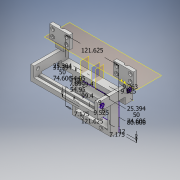
# Autodesk Inventor part: rearChassis_final
Saved by Autodesk Inventor 2018 (Build 220112000, 112)
## iProperties
Created: 2017-10-21
Part Number: rearChassis_final
Material: Generic
Document SubType Name: Modeling
Designer: Prakash
Density: 1 g/cm^3
Appearance: Default
d0: 1.500 mm
d1: 10.000 mm
d2: 18.000 mm
d3: 18.000 mm
d4: 30.000 mm
d5: 0.00 deg
d8: 10.000 mm
d9: 0.00 deg
d10: 3.588 mm
d11: 3.588 mm
d12: 34.763 mm
d13: 0.00 deg
d15: 9.763 mm
d16: 9.525 mm
d17: 8.000 mm
d22: 10.000 mm
d25: 10.000 mm
d26: 5.000 mm
d27: 70.000 mm
d28: 0.00 deg
d74: 7.000 mm
d75: 7.000 mm
d76: 7.500 mm
d77: 7.500 mm
d79: 7.500 mm
d80: 7.500 mm
d81: 3.000 mm
d89: 8.000 mm
d90: 3.175 mm
d91: 0.00 deg
d104: -68.000 mm
d117: 45.250 mm
Author: Prakash
Autodesk Inventor part; units mm, degrees
ref_plane "YZ Plane" through (0, 0, 0) normal (1, 0, 0) x (0, 1, 0)
ref_plane "XZ Plane" through (0, 0, 0) normal (0, 1, 0) x (-1, 0, 0)
ref_plane "XY Plane" through (0, 0, 0) normal (0, 0, 1) x (1, 0, 0)
sketch "Sketch1" plane through (0, 0, 0) normal (0, 0, 1) x (1, 0, 0)
  line L0 (0, 0) -> (45.5394, 0)
  line L1 (45.5394, 0) -> (45.5394, 7.5)
  line L2 (45.5394, 7.5) -> (27.5394, 7.5)
  line L3 (0, 7.5) -> (0, 0)
  line L4 (22.7697, 7.5) -> (22.7697, 9) construction
  arc A0 (18, 7.5) -> (27.5394, 7.5) centre (22.7697, 9) ccw
  circle A1 centre (22.7697, 9) radius 9 construction
  line L5 (18, 7.5) -> (0, 7.5)
  line L6 (27.5394, 7.5) -> (22.7697, 7.5) construction
  line L7 (22.7697, 7.5) -> (18, 7.5) construction
  dimension "d0" = 1.5
  dimension "d1" = 10
  dimension "d2" = 18
  dimension "d3" = 18
  constraints: 16 end point, 5 parallel, 2 centre point, 2 coincident, 2 point on circle, 1 collinear, 1 horizontal, 1 perpendicular, 1 tangent, 1 vertical
  measures "d0" distance of L4.start L4.end
  measures "d1" diameter of A0
  measures "d2" distance of L1.end L2.end
  measures "d3" diameter of A1
extrude "Extrusion1" add sketch "Sketch1" along normal blind 30
sketch "Sketch3" plane through (0, 0, 0) normal (0, 0, -1) x (-1, 0, 0)
  circle A0 centre (-22.7697, 9) radius 9 construction
  arc A1 (-27.5394, 7.5) -> (-18, 7.5) centre (-22.7697, 9) ccw projected
  arc A2 (-27.5394, 7.5) -> (-18, 7.5) centre (-22.7697, 9) ccw projected
  arc A3 (-27.5394, 7.5) -> (-18, 7.5) centre (-22.7697, 9) ccw projected
  circle A4 centre (-22.7697, 9) radius 5
  line L0 (-31.7697, 9) -> (-31.7697, 0)
  line L1 (-13.7697, 9) -> (-13.7697, 0)
  arc A5 (-22.7697, 0) -> (-13.7697, 9) centre (-22.7697, 9) ccw
  line L2 (0, 0) -> (-45.5394, 0) projected
  line L3 (-31.7697, 0) -> (-22.7697, 0)
  line L4 (-22.7697, 0) -> (-13.7697, 0)
  arc A6 (-31.7697, 9) -> (-22.7697, 0) centre (-22.7697, 9) ccw
  arc A7 (-13.7697, 9) -> (-31.7697, 9) centre (-22.7697, 9) ccw
  constraints: 8 end point, 8 point on circle, 3 centre point, 2 coincident, 2 collinear, 2 point on line, 2 tangent, 2 vertical, 1 concentric, 3 other
extrude "Extrusion2" add sketch "Sketch3" along normal blind 10
sketch "Sketch5" plane through (0, 0, -10) normal (0, 0, -1) x (-1, 0, 0)
  line L0 (-31.7697, 0) -> (-13.7697, 0) projected
  line L1 (-22.7697, 0) -> (-19.1822, 0)
  line L2 (-22.7697, 0) -> (-26.3572, 0)
  line L3 (-26.3572, 0) -> (-19.1822, 0)
  line L4 (-19.1822, 0) -> (-19.1822, 18)
  line L5 (-19.1822, 18) -> (-26.3572, 18)
  line L6 (-26.3572, 18) -> (-26.3572, 0)
  arc A0 (-13.7697, 9) -> (-31.7697, 9) centre (-22.7697, 9) ccw projected
  point P0 (0, 0)
  dimension "d10" = 3.5875
  dimension "d11" = 3.5875
  constraints: 12 end point, 2 parallel, 2 point on line, 1 horizontal, 1 midpoint, 1 perpendicular, 1 tangent
  measures "d10" distance of L1.start L1.end
  measures "d11" distance of L1.start L2.end
extrude "Extrusion3" add sketch "Sketch5" along normal blind 34.763
sketch "Sketch6" plane through (26.3572, 5.5172, -10) normal (1, 0, 0) x (0, 0, -1)
  line L0 (-10, 3.4828) -> (0, 3.4828) projected
  line L1 (0, 3.4828) -> (9.763, 3.4828) construction
  circle A0 centre (9.763, 3.4828) radius 4.7625
  circle A1 centre (9.763, 3.4828) radius 4
  point P0 (-10, -5.5172)
  dimension "d15" = 9.763
  dimension "d16" = 9.525
  dimension "d17" = 8
  constraints: 2 centre point, 2 coincident, 2 end point, 1 horizontal
  measures "d15" distance of L0.end L1.end
  measures "d16" diameter of A0
  measures "d17" diameter of A1
sketch "Sketch7" plane through (19.1822, 5.5172, -10) normal (-1, 0, 0) x (0, 0, 1)
  circle A0 centre (-9.763, 3.4828) radius 4 projected
  circle A1 centre (-9.763, 3.4828) radius 4.7625 projected
  point P0 (10, -5.5172)
sketch "Sketch8" plane through (19.1822, 5.5172, -10) normal (-1, 0, 0) x (0, 0, 1)
  line L0 (-34.763, -5.5172) -> (-34.763, 12.4828) projected
  line L1 (-34.763, 12.4828) -> (-24.763, 12.4828)
  line L2 (-24.763, 12.4828) -> (-24.763, 5.9828)
  line L3 (-24.763, 5.9828) -> (-34.763, 5.9828)
  line L4 (-34.763, 5.9828) -> (-34.763, 12.4828)
  line L5 (-34.763, -5.5172) -> (-24.763, -5.5172)
  line L6 (-24.763, -5.5172) -> (-24.763, 0.9828)
  line L7 (-24.763, 0.9828) -> (-34.763, 0.9828)
  line L8 (-34.763, 0.9828) -> (-34.763, -5.5172)
  point P0 (10, -5.5172)
  dimension "d22" = 10
  dimension "d25" = 10
  dimension "d26" = 5
  constraints: 16 end point, 4 parallel, 2 horizontal, 2 perpendicular, 1 collinear
  measures "d22" distance of L2.end L3.end
  measures "d25" distance of L6.end L7.end
  measures "d26" distance between parallel lines of L7 L3
extrude "Extrusion6" add sketch "Sketch8" along normal blind 70
sketch "Sketch11" plane through (0, 7.5, 30) normal (0, 1, 0) x (1, 0, 0)
  line L0 (13.7697, 30) -> (0, 30) projected
  line L1 (7, 30) -> (7, 0)
  line L2 (18, 0) -> (0, 0) projected
  line L3 (38.5394, 30) -> (38.5394, 0)
  line L4 (0, 30) -> (0, 0) projected
  line L5 (45.5394, 30) -> (45.5394, 0) projected
  line L6 (45.5394, 30) -> (31.7697, 30) projected
  line L7 (45.5394, 0) -> (27.5394, 0) projected
  point P0 (7, 22.5)
  point P1 (7, 7.5)
  point P2 (38.5394, 22.5)
  point P3 (38.5394, 7.5)
  dimension "d74" = 7
  dimension "d75" = 7
  dimension "d76" = 7.5
  dimension "d77" = 7.5
  dimension "d79" = 7.5
  dimension "d80" = 7.5
  constraints: 8 point on line, 4 end point, 2 vertical
  measures "d74" distance between parallel lines of L4 L1
  measures "d75" distance between parallel lines of L5 L3
  measures "d76" distance of L1.start point (7, 22.5)
  measures "d77" distance of L1.end point (7, 7.5)
  measures "d79" distance of L3.start point (38.539, 22.5)
  measures "d80" distance of L3.end point (38.539, 7.5)
hole "Hole3" at (7, 7.5, 7.5) at (7, 7.5, 22.5) at (38.5394, 7.5, 7.5) at (38.5394, 7.5, 22.5) direction (0, -1, 0) diameter 3 end up to face face through (19.7697, 0, 20) facing (0, -1, 0)
sketch "Sketch13" plane through (0, 0, 30) normal (0, -1, 0) x (1, 0, 0)
  circle A0 centre (7, -7.5) radius 1.5 projected
  circle A1 centre (38.5394, -7.5) radius 1.5 projected
  circle A2 centre (38.5394, -22.5) radius 1.5 projected
  circle A3 centre (7, -22.5) radius 1.5 projected
  line L0 (11, -9.8094) -> (7, -12.1188)
  line L1 (7, -12.1188) -> (3, -9.8094)
  line L2 (3, -9.8094) -> (3, -5.1906)
  line L3 (3, -5.1906) -> (7, -2.8812)
  line L4 (7, -2.8812) -> (11, -5.1906)
  line L5 (11, -5.1906) -> (11, -9.8094)
  line L6 (11, -20.1906) -> (11, -24.8094)
  line L7 (11, -24.8094) -> (7, -27.1188)
  line L8 (7, -27.1188) -> (3, -24.8094)
  line L9 (3, -24.8094) -> (3, -20.1906)
  line L10 (3, -20.1906) -> (7, -17.8812)
  line L11 (7, -17.8812) -> (11, -20.1906)
  line L12 (42.5394, -20.1906) -> (42.5394, -24.8094)
  line L13 (42.5394, -24.8094) -> (38.5394, -27.1188)
  line L14 (38.5394, -27.1188) -> (34.5394, -24.8094)
  line L15 (34.5394, -24.8094) -> (34.5394, -20.1906)
  line L16 (34.5394, -20.1906) -> (38.5394, -17.8812)
  line L17 (38.5394, -17.8812) -> (42.5394, -20.1906)
  line L18 (38.5394, -2.8812) -> (42.5394, -5.1906)
  line L19 (42.5394, -5.1906) -> (42.5394, -9.8094)
  line L20 (42.5394, -9.8094) -> (38.5394, -12.1188)
  line L21 (38.5394, -12.1188) -> (34.5394, -9.8094)
  line L22 (34.5394, -9.8094) -> (34.5394, -5.1906)
  line L23 (34.5394, -5.1906) -> (38.5394, -2.8812)
  line L24 (0, -30) -> (0, 0) projected
  line L25 (45.5394, -30) -> (45.5394, 0) projected
  point P0 (38.5394, -22.5)
  point P1 (38.5394, -7.5)
  dimension "d89" = 8
  constraints: 48 end point, 4 coincident, 4 parallel, 3 equal length, 52 other
  measures "d89" distance between parallel lines of L0 L3
extrude "Extrusion7" cut sketch "Sketch13" against normal blind 3.175
mirror "Mirror1" about plane through (-50.8178, 14.75, -39.763) normal (-1, 0, 0) of "Extrusion6", "Extrusion3", "Extrusion2", "Extrusion1", "Hole3", "Extrusion7"
ref_plane "Work Plane1" through (-41.6428, 5.5172, -10) normal (1, 0, 0) x (0, 0, -1)
ref_plane "Work Plane2" through (-75.5678, 5.5172, -10) normal (1, 0, 0) x (0, 0, -1)
ref_plane "Work Plane4" through (-133.4053, 9, 0) normal (0, 0, 1) x (1, 0, 0)
split body "Split1" result two bodies by plane through (-133.4053, 9, 0) normal (0, 0, 1) first body at (-120.4821, 0.5, 13.2698) (18.8465, 0.5, 16.7302)
ref_plane "Halfway plane" through (-50.8178, 5.5172, -10) normal (-1, 0, 0) x (0, 0, 1)
sketch "Sketch26" plane through (26.3572, 18, -10) normal (0, 1, 0) x (1, 0, 0)
  line L0 (0, 34.763) -> (-154.35, 34.763) projected
  line L1 (-154.35, 0) -> (-154.35, 34.763) projected
  line L2 (-121.625, 84.763) -> (-121.625, 34.763)
  line L3 (-7.175, 34.763) -> (-147.175, 34.763) projected
  line L4 (-32.725, 84.763) -> (-32.725, 34.763)
  line L5 (-32.725, 54.157) -> (-121.625, 54.157)
  line L6 (-121.625, 54.157) -> (-121.625, 66.157)
  line L7 (-121.625, 66.157) -> (-32.725, 66.157)
  line L8 (-32.725, 66.157) -> (-32.725, 54.157)
  line L9 (-32.725, 54.157) -> (-121.625, 66.157) construction
  line L10 (-121.625, 54.157) -> (-32.725, 66.157) construction
  line L11 (-121.625, 103.369) -> (-32.725, 103.369)
  line L12 (-32.725, 103.369) -> (-32.725, 115.369)
  line L13 (-32.725, 115.369) -> (-121.625, 115.369)
  line L14 (-121.625, 115.369) -> (-121.625, 103.369)
  line L15 (-121.625, 103.369) -> (-32.725, 115.369) construction
  line L16 (-32.725, 103.369) -> (-121.625, 115.369) construction
  line L17 (-121.625, 84.763) -> (-121.625, 103.369)
  line L18 (-32.725, 84.763) -> (-32.725, 103.369)
  line L19 (-121.625, 34.763) -> (-114.45, 34.763)
  line L20 (-114.45, 34.763) -> (-114.45, 115.369)
  line L21 (-114.45, 115.369) -> (-121.625, 115.369)
  line L22 (-121.625, 115.369) -> (-121.625, 34.763)
  line L23 (-32.725, 34.763) -> (-39.9, 34.763)
  line L24 (-39.9, 34.763) -> (-39.9, 115.369)
  line L25 (-39.9, 115.369) -> (-32.725, 115.369)
  line L26 (-32.725, 115.369) -> (-32.725, 34.763)
  line L27 (-121.625, 103.369) -> (-32.725, 103.369)
  line L28 (-32.725, 103.369) -> (-32.725, 115.369)
  line L29 (-32.725, 115.369) -> (-121.625, 115.369)
  line L30 (-121.625, 115.369) -> (-121.625, 103.369)
  point P0 (-26.3572, -10)
  point P1 (-77.175, 60.157)
  point P2 (-77.175, 109.369)
  point P3 (-99.4, 60.157)
  point P4 (-54.95, 60.157)
  point P5 (-54.95, 109.369)
  point P6 (-99.4, 109.369)
  dimension "d149" = 12
  dimension "d150" = 12
  dimension "d153" = 121.625
  dimension "d154" = 7.175
  dimension "d155" = 7.175
  dimension "d156" = 7.688
  dimension "d157" = 80.606
  dimension "d158" = 31.394
  dimension "d159" = 121.625
  dimension "d160" = 50
  dimension "d161" = 74.606
  dimension "d162" = 99.4
  dimension "d163" = 25.394
  dimension "d164" = 99.4
  dimension "d165" = 74.606
  dimension "d166" = 54.95
  dimension "d167" = 25.394
  dimension "d168" = 54.95
  dimension "d169" = 50
  constraints: 56 end point, 15 parallel, 5 perpendicular, 4 midpoint, 4 point on line, 3 horizontal, 1 collinear, 1 vertical
  measures "d149" distance of L5.end L6.end
  measures "d150" distance of L12.end L11.end
  measures "d153" distance between parallel lines of L18 L1
  measures "d154" distance of L21.end L20.end
  measures "d155" distance of L24.end L25.end
  measures "d156" angle of L3 L15
  measures "d157" distance between parallel lines of L3 L13
  measures "d158" distance between parallel lines of L3 L7
  measures "d159" distance between parallel lines of L8 L1
  measures "d160" distance from line of L4.start L3
  measures "d161" distance from line of point (-54.95, 109.369) L3
  measures "d162" distance from line of point (-54.95, 109.369) L1
  measures "d163" distance from line of point (-54.95, 60.157) L3
  measures "d164" distance from line of point (-54.95, 60.157) L1
  measures "d165" distance from line of point (-99.4, 109.369) L3
  measures "d166" distance from line of point (-99.4, 109.369) L1
  measures "d167" distance from line of point (-99.4, 60.157) L3
  measures "d168" distance from line of point (-99.4, 60.157) L1
  measures "d169" distance from line of L2.start L3
extrude "Extrusion14" add sketch "Sketch26" against normal up to surface (18 mm away) contours L0 L24 L5 L4 | L5 L24 L7 L4 | L0 L2 L5 L20 | L5 L20 L7 L24 | L7 L24 L11 L18 L4 | L5 L2 L7 L20 | L7 L2 L17 L11 L20 | L24 L13 L12 L11 | L11 L20 L13 L24 | L11 L14 L13 L20 bodies 3
hole "Hole5" at (-28.5928, 18, -70.157) at (-28.5928, 18, -119.369) at (-73.0428, 18, -70.157) at (-73.0428, 18, -119.369) direction (0, -1, 0) diameter 3 end up to face face through (-65.6345, 0, -38.0963) facing (0, -1, 0) bodies 3
sketch "Sketch27" plane through (13.7697, 0, 0) normal (0, -1, 0) x (1, 0, 0)
  line L0 (-2.7697, 9.8094) -> (-2.7697, 5.1906) projected
  line L1 (-6.7697, 12.1188) -> (-2.7697, 9.8094) projected
  line L2 (-13.7697, 0) -> (31.7697, 0) projected
  line L3 (31.7697, 0) -> (31.7697, 30) projected
  line L4 (-13.7697, 30) -> (31.7697, 30) projected
  line L5 (-13.7697, 0) -> (-13.7697, 30) projected
  line L6 (20.7697, 24.8094) -> (24.7697, 27.1188) projected
  line L7 (24.7697, 27.1188) -> (28.7697, 24.8094) projected
  line L8 (28.7697, 24.8094) -> (28.7697, 20.1906) projected
  line L9 (28.7697, 20.1906) -> (24.7697, 17.8812) projected
  line L10 (24.7697, 17.8812) -> (20.7697, 20.1906) projected
  line L11 (20.7697, 20.1906) -> (20.7697, 24.8094) projected
  line L12 (-6.7697, 12.1188) -> (-2.7697, 9.8094) projected
  line L13 (-2.7697, 9.8094) -> (-2.7697, 5.1906) projected
  line L14 (-2.7697, 5.1906) -> (-6.7697, 2.8812) projected
  line L15 (-6.7697, 2.8812) -> (-10.7697, 5.1906) projected
  line L16 (-10.7697, 5.1906) -> (-10.7697, 9.8094) projected
  line L17 (-10.7697, 9.8094) -> (-6.7697, 12.1188) projected
  line L18 (-2.7697, 24.8094) -> (-2.7697, 20.1906) projected
  line L19 (-2.7697, 20.1906) -> (-6.7697, 17.8812) projected
  line L20 (-6.7697, 17.8812) -> (-10.7697, 20.1906) projected
  line L21 (-10.7697, 20.1906) -> (-10.7697, 24.8094) projected
  line L22 (-10.7697, 24.8094) -> (-6.7697, 27.1188) projected
  line L23 (-6.7697, 27.1188) -> (-2.7697, 24.8094) projected
  line L24 (24.7697, 12.1188) -> (28.7697, 9.8094) projected
  line L25 (28.7697, 9.8094) -> (28.7697, 5.1906) projected
  line L26 (28.7697, 5.1906) -> (24.7697, 2.8812) projected
  line L27 (24.7697, 2.8812) -> (20.7697, 5.1906) projected
  line L28 (20.7697, 5.1906) -> (20.7697, 9.8094) projected
  line L29 (20.7697, 9.8094) -> (24.7697, 12.1188) projected
  circle A0 centre (-42.3625, -70.157) radius 1.5 projected
  line L30 (-44.6719, -74.157) -> (-46.9813, -70.157)
  line L31 (-46.9813, -70.157) -> (-44.6719, -66.157)
  line L32 (-44.6719, -66.157) -> (-40.0531, -66.157)
  line L33 (-40.0531, -66.157) -> (-37.7437, -70.157)
  line L34 (-37.7437, -70.157) -> (-40.0531, -74.157)
  line L35 (-40.0531, -74.157) -> (-44.6719, -74.157)
  circle A1 centre (-86.8125, -70.157) radius 1.5 projected
  line L36 (-91.4313, -70.157) -> (-89.1219, -66.157)
  line L37 (-89.1219, -66.157) -> (-84.5031, -66.157)
  line L38 (-84.5031, -66.157) -> (-82.1937, -70.157)
  line L39 (-82.1937, -70.157) -> (-84.5031, -74.157)
  line L40 (-84.5031, -74.157) -> (-89.1219, -74.157)
  line L41 (-89.1219, -74.157) -> (-91.4313, -70.157)
  circle A2 centre (-86.8125, -119.369) radius 1.5 projected
  line L42 (-91.4313, -119.369) -> (-89.1219, -115.369)
  line L43 (-89.1219, -115.369) -> (-84.5031, -115.369)
  line L44 (-84.5031, -115.369) -> (-82.1937, -119.369)
  line L45 (-82.1937, -119.369) -> (-84.5031, -123.369)
  line L46 (-84.5031, -123.369) -> (-89.1219, -123.369)
  line L47 (-89.1219, -123.369) -> (-91.4313, -119.369)
  circle A3 centre (-42.3625, -119.369) radius 1.5 projected
  line L48 (-46.9813, -119.369) -> (-44.6719, -115.369)
  line L49 (-44.6719, -115.369) -> (-40.0531, -115.369)
  line L50 (-40.0531, -115.369) -> (-37.7437, -119.369)
  line L51 (-37.7437, -119.369) -> (-40.0531, -123.369)
  line L52 (-40.0531, -123.369) -> (-44.6719, -123.369)
  line L53 (-44.6719, -123.369) -> (-46.9813, -119.369)
  point P0 (-42.3625, -70.157)
  point P1 (-86.8125, -70.157)
  point P2 (-86.8125, -119.369)
  point P3 (-42.3625, -119.369)
  constraints: 48 end point, 4 coincident, 4 equal length, 4 horizontal, 52 other
extrude "Extrusion15" cut sketch "Sketch27" against normal blind 3.175 contours L30 L31 L32 L33 L34 L35 | L36 L37 L38 L39 L40 L41 | L42 L43 L44 L45 L46 L47 | L48 L49 L50 L51 L52 L53 bodies 3
sketch "Sketch30" plane through (13.7697, 0, 0) normal (0, -1, 0) x (1, 0, 0)
  line L0 (12.5875, -10) -> (12.5875, -44.763) projected
  line L1 (5.4125, -10) -> (12.5875, -10)
  line L2 (12.5875, -10) -> (12.5875, -29.526)
  line L3 (12.5875, -29.526) -> (5.4125, -29.526)
  line L4 (5.4125, -29.526) -> (5.4125, -10)
  line L5 (-141.7625, -10) -> (-134.5875, -10) projected
  line L6 (-141.7625, -10) -> (-134.5875, -10)
  line L7 (-134.5875, -10) -> (-134.5875, -29.526)
  line L8 (-134.5875, -29.526) -> (-141.7625, -29.526)
  line L9 (-141.7625, -29.526) -> (-141.7625, -10)
  point P0 (-13.7697, 0)
  dimension "d181" = 19.526
  dimension "d182" = 19.526
  constraints: 16 end point, 5 equal length, 2 perpendicular, 1 horizontal
  measures "d181" distance of L0.start L2.end
  measures "d182" distance of L5.end L7.end
extrude "Extrusion16" add sketch "Sketch30" along normal blind 62.5 bodies 3
sketch "Sketch31" plane through (26.3572, 5.5172, -10) normal (1, 0, 0) x (0, 0, -1)
  line L0 (19.526, -68.0172) -> (0, -68.0172) construction
  line L1 (9.763, -68.0172) -> (9.763, -59.0172) construction
  circle A0 centre (9.763, -59.0172) radius 4.7625
  circle A1 centre (9.763, -59.0172) radius 4
  point P0 (-10, -5.5172)
  dimension "d185" = 9
  dimension "d186" = 9.525
  dimension "d187" = 8
  constraints: 2 centre point, 2 coincident, 2 end point, 1 midpoint, 1 vertical
  measures "d185" distance of L1.start L1.end
  measures "d186" diameter of A0
  measures "d187" diameter of A1
extrude "Extrusion17" cut sketch "Sketch31" against normal up to surface (7.175 mm away) contours A1 bodies 3
extrude "Extrusion18" cut sketch "Sketch31" against normal blind 3.175 bodies 3
mirror "Mirror4" about plane through (-50.8178, 5.5172, -10) normal (-1, 0, 0) of "Extrusion18", "Extrusion17" bodies 3
sketch "Sketch35" plane through (19.1822, 6.5, -34.763) normal (0, 1, 0) x (1, 0, 0)
  line L0 (-94.5344, 88.606) -> (-96.8438, 84.606) projected
  line L1 (-96.8438, 84.606) -> (-94.5344, 80.606) projected
  line L2 (-94.5344, 80.606) -> (-89.9156, 80.606) projected
  line L3 (-89.9156, 80.606) -> (-87.6062, 84.606) projected
  line L4 (-87.6062, 84.606) -> (-89.9156, 88.606) projected
  line L5 (-89.9156, 88.606) -> (-94.5344, 88.606) projected
  line L6 (-45.4656, 39.394) -> (-50.0844, 39.394) projected
  line L7 (-50.0844, 39.394) -> (-52.3938, 35.394) projected
  line L8 (-52.3938, 35.394) -> (-50.0844, 31.394) projected
  line L9 (-50.0844, 31.394) -> (-45.4656, 31.394) projected
  line L10 (-45.4656, 31.394) -> (-43.1562, 35.394) projected
  line L11 (-43.1562, 35.394) -> (-45.4656, 39.394) projected
  line L12 (-94.5344, 39.394) -> (-96.8438, 35.394) projected
  line L13 (-96.8438, 35.394) -> (-94.5344, 31.394) projected
  line L14 (-94.5344, 31.394) -> (-89.9156, 31.394) projected
  line L15 (-89.9156, 31.394) -> (-87.6062, 35.394) projected
  line L16 (-87.6062, 35.394) -> (-89.9156, 39.394) projected
  line L17 (-89.9156, 39.394) -> (-94.5344, 39.394) projected
  line L18 (-50.0844, 88.606) -> (-52.3938, 84.606) projected
  line L19 (-52.3938, 84.606) -> (-50.0844, 80.606) projected
  line L20 (-50.0844, 80.606) -> (-45.4656, 80.606) projected
  line L21 (-45.4656, 80.606) -> (-43.1562, 84.606) projected
  line L22 (-43.1562, 84.606) -> (-45.4656, 88.606) projected
  line L23 (-45.4656, 88.606) -> (-50.0844, 88.606) projected
  line L24 (7.175, -5.237) -> (0, -5.237) projected
  line L25 (0, -5.237) -> (0, 0) projected
  line L26 (0, 0) -> (-140, 0) projected
  line L27 (-140, -5.237) -> (-140, 0) projected
  line L28 (-140, -5.237) -> (-147.175, -5.237) projected
  line L29 (-147.175, -5.237) -> (-147.175, 10) projected
  line L30 (-114.45, 10) -> (-147.175, 10) projected
  line L31 (-114.45, 90.606) -> (-114.45, 10) projected
  line L32 (-25.55, 90.606) -> (-114.45, 90.606) projected
  line L33 (-25.55, 10) -> (-25.55, 90.606) projected
  line L34 (7.175, 10) -> (-25.55, 10) projected
  line L35 (7.175, -5.237) -> (7.175, 10) projected
  line L36 (-32.725, 41.394) -> (-107.275, 41.394) projected
  line L37 (-32.725, 78.606) -> (-32.725, 41.394) projected
  line L38 (-107.275, 78.606) -> (-32.725, 78.606) projected
  line L39 (-107.275, 41.394) -> (-107.275, 78.606) projected
  line L40 (-32.725, 29.394) -> (-32.725, 10) projected
  line L41 (-107.275, 29.394) -> (-32.725, 29.394) projected
  line L42 (-107.275, 10) -> (-107.275, 29.394) projected
  line L43 (-32.725, 10) -> (-107.275, 10) projected
  line L44 (0, 0) -> (0, 10)
  line L45 (0, 10) -> (-140, 10)
  line L46 (-140, 10) -> (-140, 0)
  line L47 (-140, 0) -> (0, 0)
  point P0 (-19.1822, -34.763)
  dimension "d192" = 140
  constraints: 8 end point, 2 parallel, 2 perpendicular, 1 point on line
  measures "d192" distance between parallel lines of L44 L46
extrude "Extrusion19" add sketch "Sketch35" along normal up to next contours L26 L46 L30 L45 L43 L34 L44 bodies 3
sketch "Sketch36" plane through (26.3572, 0, -29.526) normal (0, 0, -1) x (-1, 0, 0)
  line L0 (0, 0) -> (7.175, 0) projected
  line L1 (0, 0) -> (0, -62.5) projected
  line L2 (7.175, -62.5) -> (0, -62.5) projected
  line L3 (7.175, 0) -> (7.175, -62.5) projected
  line L4 (147.175, 0) -> (154.35, 0) projected
  line L5 (147.175, 0) -> (147.175, -62.5) projected
  line L6 (154.35, -62.5) -> (147.175, -62.5) projected
  line L7 (154.35, 0) -> (154.35, -62.5) projected
  line L8 (7.175, -62.5) -> (0, -62.5)
  line L9 (0, -62.5) -> (0, -44.5)
  line L10 (0, -44.5) -> (7.175, -44.5)
  line L11 (7.175, -44.5) -> (7.175, -62.5)
  point P0 (26.3572, 0)
  dimension "d195" = 18
  constraints: 8 end point, 2 parallel, 1 horizontal, 1 perpendicular
  measures "d195" distance of L1.end L9.end
extrude "Extrusion20" add sketch "Sketch36" along normal blind 14 contours L10 L3 L2 L1 bodies 3
sketch "Sketch37" plane through (19.1822, 5.5172, -10) normal (-1, 0, 0) x (0, 0, 1)
  line L0 (-24.763, 12.4828) -> (-24.763, -5.5172) projected
  line L1 (-19.526, -5.5172) -> (-24.763, -5.5172) projected
  line L2 (-19.526, -5.5172) -> (-19.526, -50.0172) projected
  line L3 (-19.526, -50.0172) -> (-33.526, -50.0172) projected
  line L4 (-33.526, -68.0172) -> (-33.526, -50.0172) projected
  line L5 (0, -68.0172) -> (-33.526, -68.0172) projected
  line L6 (0, -5.5172) -> (0, -68.0172) projected
  line L7 (0, 0) -> (0, -5.5172) projected
  line L8 (0, 0) -> (0, 6.9656) projected
  line L9 (0, 11.7369) -> (0, 6.9656) projected
  line L10 (0, 11.7369) -> (0, 12.4828) projected
  line L11 (0, 12.4828) -> (-24.763, 12.4828) projected
  circle A0 centre (-9.763, -59.0172) radius 4 projected
  line L12 (-33.526, -50.0172) -> (-23.526, -50.0172)
  line L13 (-23.526, -50.0172) -> (-23.526, -56.5172)
  line L14 (-23.526, -56.5172) -> (-33.526, -56.5172)
  line L15 (-33.526, -56.5172) -> (-33.526, -50.0172)
  line L16 (-33.526, -68.0172) -> (-23.526, -68.0172)
  line L17 (-23.526, -68.0172) -> (-23.526, -61.5172)
  line L18 (-23.526, -61.5172) -> (-33.526, -61.5172)
  line L19 (-33.526, -61.5172) -> (-33.526, -68.0172)
  point P0 (10, -5.5172)
  point P1 (-19.526, -5.5172)
  dimension "d198" = 10
  dimension "d199" = 10
  dimension "d200" = 5
  constraints: 16 end point, 4 parallel, 2 perpendicular, 2 point on line, 1 collinear
  measures "d198" distance of L3.end L12.end
  measures "d199" distance of L4.start L16.end
  measures "d200" distance between parallel lines of L18 L14
extrude "Extrusion21" add sketch "Sketch37" along normal up to surface (70 mm away) contours L13 L14 L4 L3 | L18 L17 L5 L4 bodies 3
mirror "Mirror5" about plane through (-50.8178, 5.5172, -10) normal (-1, 0, 0) of "Extrusion21", "Extrusion20" bodies 3
body "Solid2"
body "Solid3"
